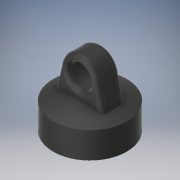
# Autodesk Inventor part: タミヤダンパー部品1
Saved by Autodesk Inventor 2020.1 (Build 241239000, 239)
## iProperties
Created: 2018-09-17
Part Number: タミヤダンパー部品1
Material: アセタール樹脂、黒
Document SubType Name: Modeling
Designer: 杉本　賢二郎
Density: 1.425 g/cm^3
Appearance: 滑らか - 黒
Author: 杉本　賢二郎
Autodesk Inventor part; units mm, degrees
ref_plane "YZ Plane" through (0, 0, 0) normal (1, 0, 0) x (0, 1, 0)
ref_plane "XZ Plane" through (0, 0, 0) normal (0, 1, 0) x (-1, 0, 0)
ref_plane "XY Plane" through (0, 0, 0) normal (0, 0, 1) x (1, 0, 0)
sketch "スケッチ1" plane through (0, 0, 0) normal (0, 1, 0) x (-1, 0, 0)
  circle A0 centre (0, 0) radius 7.875
  dimension "d0" = 15.75
  constraints: 1 centre point, 1 coincident
  measures "d0" diameter of A0
extrude "押し出し1" add sketch "スケッチ1" along normal blind 5.6
sketch "スケッチ2" plane through (0, 0, 0) normal (0, 0, 1) x (1, 0, 0)
  line L0 (7.875, 5.6) -> (-7.875, 5.6)
  circle A0 centre (0, 11.033601) radius 2.5
  arc A1 (3.89748, 11.933405) -> (-3.89748, 11.933405) centre (0, 11.033601) ccw
  line L1 (3.89748, 11.933405) -> (5.359662, 5.6)
  line L2 (-3.89748, 11.933405) -> (-5.359662, 5.6)
  line L3 (0, 11.033601) -> (0.809241, 11.033601)
  point P0 (0, 0)
  point P1 (0, 0)
  dimension "d3" = 5
  dimension "d4" = 1.5
  dimension "d5" = 103
  dimension "d6" = 103
  dimension "d7" = 6.5
  constraints: 8 end point, 2 centre point, 2 point on circle, 2 point on line, 2 tangent, 1 horizontal, 1 vertical alignment
  measures "d3" diameter of A0
  measures "d4" radial gap between concentric circles of A0 A1
  measures "d5" angle of L3 L1
  measures "d6" angle of L2 L3
  measures "d7" distance of L1.start L1.end
extrude "押し出し2" add sketch "スケッチ2" along normal mid plane 5
sketch "スケッチ3" plane through (0, 0, 0) normal (0, 0, 1) x (1, 0, 0)
  line L0 (7.875, 5.6) -> (-7.875, 5.6)
  line L1 (0, 5.6) -> (0, 7.215649)
  arc A0 (7.875, 5.6) -> (0, 7.215649) centre (0, -12.784351) ccw
  line L2 (0, -18.347942) -> (0, 20.597192)
  point P0 (0, 0)
  point P1 (0, 0)
  dimension "d10" = 20
  constraints: 5 end point, 2 point on circle, 1 centre point, 1 midpoint, 1 vertical, 1 other
  measures "d10" radius of A0
revolve "回転1" add sketch "スケッチ3" angle 360 about axis through (0, -10, 0) along (0, 1, 0)
sketch "スケッチ4" plane through (0, 0, 0) normal (0, 1, 0) x (-1, 0, 0)
  circle A0 centre (0, 0) radius 5.5
  dimension "d12" = 11
  constraints: 1 centre point, 1 coincident
  measures "d12" diameter of A0
extrude "押し出し3" cut sketch "スケッチ4" along normal blind 4
fillet "フィレット1" radius 1 8 edges at (-4.5397, 9.1518, 2.5) (4.5397, 9.1518, 2.5) (0, 15.0336, 2.5) (-2.5, 11.0336, 2.5) (0, 15.0336, -2.5) (4.5397, 9.1518, -2.5) (-4.5397, 9.1518, -2.5) (-2.5, 11.0336, -2.5)
equation "\"d6\" = d5"
